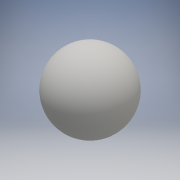
# Autodesk Inventor part: Ball
Saved by Autodesk Inventor 2016 (Build 200138000, 138)
## iProperties
Created: 2016-10-31
Part Number: Ball
Material: Generic
Document SubType Name: Modeling
Designer: mattc
Density: 1 g/cm^3
Appearance: Default
Author: mattc
Autodesk Inventor part; units mm, degrees
ref_plane "YZ Plane" through (0, 0, 0) normal (1, 0, 0) x (0, 1, 0)
ref_plane "XZ Plane" through (0, 0, 0) normal (0, 1, 0) x (-1, 0, 0)
ref_plane "XY Plane" through (0, 0, 0) normal (0, 0, 1) x (1, 0, 0)
sketch "Sketch1" plane through (0, 0, 0) normal (0, 0, 1) x (1, 0, 0)
  line L0 (0, 28.575) -> (0, -28.575)
  arc A0 (0, -28.575) -> (0, 28.575) centre (0, 0) ccw
  dimension "d5" = 28.575
  dimension "d6" = 28.575
  dimension "d9" = 57.15
  constraints: 2 end point, 2 point on circle, 2 vertical, 1 centre point
  measures "d5" radius of A0
  measures "d6" distance of point (0, 0) L0.start
  measures "d9" distance of L0.start L0.end
revolve "Revolution1" add sketch "Sketch1" angle 360 about axis through (0, 28.575, 0) along (0, -1, 0)
equation "\"d5\" = 0.5 * d9"
equation "\"d6\" = 0.5 * d9"
body "Solid1"
